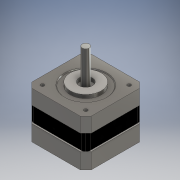
# Autodesk Inventor part: SmallStepper
Saved by Autodesk Inventor 2016 (Build 200138000, 138)
## iProperties
Created: 2016-05-03
Part Number: SmallStepper
Material: Stainless Steel
Document SubType Name: Modeling
Designer: Kurtis
Density: 8 g/cm^3
Appearance: Semi-Polished
Author: Kurtis
Autodesk Inventor part; units mm, degrees
ref_plane "YZ Plane" through (0, 0, 0) normal (1, 0, 0) x (0, 1, 0)
ref_plane "XZ Plane" through (0, 0, 0) normal (0, 1, 0) x (-1, 0, 0)
sketch "Sketch1" plane through (0, 0, 0) normal (0, 0, 1) x (1, 0, 0)
  line L0 (-17.1838, -21) -> (17.1838, -21)
  line L1 (21, -17.1838) -> (21, 17.1838)
  line L2 (17.1838, 21) -> (-17.1838, 21)
  line L3 (-21, 17.1838) -> (-21, -17.1838)
  line L4 (-21, -21) -> (21, 21) construction
  line L5 (21, -21) -> (-21, 21) construction
  line L6 (0, 0) -> (19.0919, -19.0919) construction
  line L7 (0, 0) -> (-19.0919, -19.0919) construction
  line L8 (0, 0) -> (-19.0919, 19.0919) construction
  line L9 (0, 0) -> (19.0919, 19.0919) construction
  line L10 (19.0919, -19.0919) -> (17.1838, -21)
  line L11 (19.0919, -19.0919) -> (21, -17.1838)
  line L12 (-19.0919, -19.0919) -> (-21, -17.1838)
  line L13 (-19.0919, -19.0919) -> (-17.1838, -21)
  line L14 (-19.0919, 19.0919) -> (-21, 17.1838)
  line L15 (-19.0919, 19.0919) -> (-17.1838, 21)
  line L16 (19.0919, 19.0919) -> (21, 17.1838)
  line L17 (19.0919, 19.0919) -> (17.1838, 21)
  line L18 (-15.375, 15.375) -> (15.375, 15.375) construction
  line L19 (15.375, 15.375) -> (15.375, -15.375) construction
  line L20 (15.375, -15.375) -> (-15.375, -15.375) construction
  line L21 (-15.375, -15.375) -> (-15.375, 15.375) construction
  line L22 (-15.375, 15.375) -> (15.375, -15.375) construction
  line L23 (15.375, 15.375) -> (-15.375, -15.375) construction
  circle A0 centre (15.375, 15.375) radius 1.25
  circle A1 centre (-15.375, 15.375) radius 1.25
  circle A2 centre (-15.375, -15.375) radius 1.25
  circle A3 centre (15.375, -15.375) radius 1.25
  dimension "d0" = 42
  dimension "d1" = 42
  dimension "d2" = 27
  dimension "d3" = 27
  dimension "d4" = 27
  dimension "d5" = 27
  dimension "d18" = 34.3675
  dimension "d19" = 30.75
  dimension "d20" = 30.75
  dimension "d21" = 2.5
  dimension "d22" = 2.5
  dimension "d23" = 2.5
  dimension "d24" = 2.5
  constraints: 48 end point, 8 point on line, 6 parallel, 5 perpendicular, 4 centre point, 4 coincident, 4 collinear, 4 midpoint, 2 horizontal
  measures "d0" distance of L5.end L4.end
  measures "d1" distance of L4.end L5.start
  measures "d2" distance of L6.start L6.end
  measures "d3" distance of L6.start L7.end
  measures "d4" distance of L6.start L8.end
  measures "d5" distance of L6.start L9.end
  measures "d18" distance of L2.start L2.end
  measures "d19" distance of L19.end L20.end
  measures "d20" distance of L18.end L19.end
  measures "d21" diameter of A0
  measures "d22" diameter of A1
  measures "d23" diameter of A2
  measures "d24" diameter of A3
extrude "Body" add sketch "Sketch1" along normal blind 33
sketch "Sketch2" plane through (0, 0, 33) normal (0, 0, 1) x (1, 0, 0)
  circle A0 centre (0, 0) radius 11
  dimension "d27" = 22
  constraints: 1 centre point, 1 coincident
  measures "d27" diameter of A0
extrude "Raised" add sketch "Sketch2" along normal blind 2
sketch "Sketch3" plane through (0, 0, 35) normal (0, 0, 1) x (1, 0, 0)
  circle A0 centre (0, 0) radius 2.5
  dimension "d30" = 5
  constraints: 1 centre point, 1 coincident
  measures "d30" diameter of A0
extrude "Axle" add sketch "Sketch3" along normal blind 22
sketch "Sketch4" plane through (0, 0, 35) normal (0, 0, 1) x (1, 0, 0)
  circle A0 centre (0, 0) radius 2.5
  circle A1 centre (0, 0) radius 4.75
  circle A2 centre (0, 0) radius 11
  circle A3 centre (0, 0) radius 15
  dimension "d33" = 9.5
  dimension "d34" = 30
  constraints: 4 centre point, 4 coincident
  measures "d33" diameter of A1
  measures "d34" diameter of A3
extrude "Face Indent" cut sketch "Sketch4" against normal blind 2.5
chamfer "Indent Chamf" distance 0.5 angle 45 1 edges at (-15, 0, 32.5)
sketch "Sketch5" plane through (-17.1838, 21, 0) normal (0, 1, 0) x (1, 0, 0)
  line L0 (17.1838, 0) -> (25.1838, 0)
  line L1 (34.3675, 0) -> (0, 0) projected
  line L2 (25.1838, 0) -> (25.1838, -11.25)
  line L3 (25.1838, -11.25) -> (9.1838, -11.25)
  line L4 (9.1838, -11.25) -> (9.1838, 0)
  line L5 (17.1838, 0) -> (9.1838, 0)
  dimension "d40" = 8
  dimension "d41" = 11.25
  dimension "d42" = 16
  constraints: 10 end point, 3 perpendicular, 2 point on line, 1 collinear
  measures "d40" distance of L0.start L0.end
  measures "d41" distance of L0.end L2.end
  measures "d42" distance of L2.end L3.end
extrude "Power Base" add sketch "Sketch5" along normal blind 3.75
sketch "Sketch6" plane through (-17.1838, 24.75, 0) normal (0, 1, 0) x (1, 0, 0)
  line L0 (25.1838, -11.25) -> (9.1838, -11.25) projected
  line L1 (25.1838, -11.25) -> (25.1838, -4.85)
  line L2 (25.1838, 0) -> (25.1838, -11.25) projected
  line L3 (25.1838, -4.85) -> (9.1838, -4.85)
  line L4 (9.1838, -11.25) -> (9.1838, 0) projected
  line L5 (9.1838, -4.85) -> (9.1838, -11.25)
  line L6 (9.1838, -11.25) -> (25.1838, -11.25)
  line L7 (25.1838, -8.05) -> (24.1838, -8.05) construction
  line L8 (17.1838, -4.85) -> (17.1838, -5.85) construction
  line L9 (9.1838, 0) -> (9.1838, -11.25) construction
  line L10 (9.1838, -8.05) -> (10.1838, -8.05) construction
  line L11 (17.1838, -11.25) -> (17.1838, -10.75) construction
  line L12 (17.1838, -10.75) -> (21.1838, -10.75) construction
  line L13 (17.1838, -10.75) -> (13.1838, -10.75) construction
  line L14 (24.1838, -5.85) -> (10.1838, -5.85)
  line L15 (10.1838, -5.85) -> (10.1838, -10.75)
  line L16 (10.1838, -10.75) -> (13.1838, -10.75)
  line L17 (24.1838, -5.85) -> (24.1838, -10.75)
  line L18 (21.1838, -10.75) -> (24.1838, -10.75)
  line L19 (10.1838, -8.3) -> (24.1838, -8.3) construction
  line L20 (24.1838, -8.3) -> (22.6123, -8.3) construction
  line L21 (22.6123, -8.3) -> (22.1123, -8.3)
  line L22 (22.1123, -8.3) -> (20.5409, -8.3) construction
  line L23 (20.5409, -8.3) -> (20.0409, -8.3)
  line L24 (20.0409, -8.3) -> (18.4695, -8.3) construction
  line L25 (18.4695, -8.3) -> (17.9695, -8.3)
  line L26 (17.9695, -8.3) -> (16.3981, -8.3) construction
  line L27 (16.3981, -8.3) -> (15.8981, -8.3)
  line L28 (15.8981, -8.3) -> (14.3266, -8.3) construction
  line L29 (14.3266, -8.3) -> (13.8266, -8.3)
  line L30 (13.8266, -8.3) -> (12.2552, -8.3) construction
  line L31 (12.2552, -8.3) -> (11.7552, -8.3)
  line L32 (11.7552, -8.3) -> (10.1838, -8.3) construction
  line L33 (22.6123, -8.05) -> (22.1123, -8.05)
  line L34 (22.1123, -8.05) -> (22.1123, -8.55)
  line L35 (22.1123, -8.55) -> (22.6123, -8.55)
  line L36 (22.6123, -8.55) -> (22.6123, -8.05)
  line L37 (22.6123, -8.05) -> (22.1123, -8.55) construction
  line L38 (22.1123, -8.05) -> (22.6123, -8.55) construction
  line L39 (20.5409, -8.05) -> (20.0409, -8.05)
  line L40 (20.0409, -8.05) -> (20.0409, -8.55)
  line L41 (20.0409, -8.55) -> (20.5409, -8.55)
  line L42 (20.5409, -8.55) -> (20.5409, -8.05)
  line L43 (20.5409, -8.05) -> (20.0409, -8.55) construction
  line L44 (20.0409, -8.05) -> (20.5409, -8.55) construction
  line L45 (18.4695, -8.05) -> (17.9695, -8.05)
  line L46 (17.9695, -8.05) -> (17.9695, -8.55)
  line L47 (17.9695, -8.55) -> (18.4695, -8.55)
  line L48 (18.4695, -8.55) -> (18.4695, -8.05)
  line L49 (18.4695, -8.05) -> (17.9695, -8.55) construction
  line L50 (17.9695, -8.05) -> (18.4695, -8.55) construction
  line L51 (16.3981, -8.05) -> (15.8981, -8.05)
  line L52 (15.8981, -8.05) -> (15.8981, -8.55)
  line L53 (15.8981, -8.55) -> (16.3981, -8.55)
  line L54 (16.3981, -8.55) -> (16.3981, -8.05)
  line L55 (16.3981, -8.05) -> (15.8981, -8.55) construction
  line L56 (15.8981, -8.05) -> (16.3981, -8.55) construction
  line L57 (14.3266, -8.05) -> (13.8266, -8.05)
  line L58 (13.8266, -8.05) -> (13.8266, -8.55)
  line L59 (13.8266, -8.55) -> (14.3266, -8.55)
  line L60 (14.3266, -8.55) -> (14.3266, -8.05)
  line L61 (14.3266, -8.05) -> (13.8266, -8.55) construction
  line L62 (13.8266, -8.05) -> (14.3266, -8.55) construction
  line L63 (12.2552, -8.05) -> (11.7552, -8.05)
  line L64 (11.7552, -8.05) -> (11.7552, -8.55)
  line L65 (11.7552, -8.55) -> (12.2552, -8.55)
  line L66 (12.2552, -8.55) -> (12.2552, -8.05)
  line L67 (12.2552, -8.05) -> (11.7552, -8.55) construction
  line L68 (11.7552, -8.05) -> (12.2552, -8.55) construction
  line L69 (13.1838, -10.75) -> (13.1838, -11.25)
  line L70 (21.1838, -10.75) -> (21.1838, -11.25)
  line L71 (9.1838, -11.25) -> (25.1838, -11.25) projected
  point P0 (17.1838, 0)
  point P1 (22.3623, -8.3)
  point P2 (20.2909, -8.3)
  point P3 (18.2195, -8.3)
  point P4 (16.1481, -8.3)
  point P5 (14.0766, -8.3)
  point P6 (12.0052, -8.3)
  dimension "d45" = 6.4
  dimension "d48" = 1
  dimension "d49" = 1
  dimension "d50" = 1
  dimension "d51" = 0.5
  dimension "d52" = 4
  dimension "d53" = 4
  dimension "d59" = 1.5714
  dimension "d60" = 0.5
  dimension "d61" = 1.5714
  dimension "d62" = 0.5
  dimension "d63" = 1.5714
  dimension "d64" = 0.5
  dimension "d65" = 1.5714
  dimension "d66" = 0.5
  dimension "d67" = 1.5714
  dimension "d68" = 0.5
  dimension "d69" = 1.5714
  dimension "d70" = 0.5
  dimension "d71" = 0.5
  dimension "d72" = 0.5
  dimension "d73" = 0.5
  dimension "d74" = 0.5
  dimension "d75" = 0.5
  dimension "d76" = 0.5
  dimension "d77" = 0.5
  dimension "d78" = 0.5
  dimension "d79" = 0.5
  dimension "d80" = 0.5
  dimension "d81" = 2.5714
  dimension "d82" = 3.2
  dimension "d83" = 1
  dimension "d84" = 3.2
  dimension "d85" = 3.2
  constraints: 132 end point, 22 midpoint, 18 parallel, 11 perpendicular, 7 horizontal, 6 point on line, 3 collinear, 3 vertical, 15 other
  measures "d45" distance of L0.start L1.end
  measures "d48" distance of L7.start L7.end
  measures "d49" distance of L8.start L8.end
  measures "d50" distance of L10.start L10.end
  measures "d51" distance of L11.start L11.end
  measures "d52" distance of L11.end L12.end
  measures "d53" distance of L11.end L13.end
  measures "d59" distance of L20.start L20.end
  measures "d60" distance of L20.end L21.end
  measures "d61" distance of L21.end L22.end
  measures "d62" distance of L22.end L23.end
  measures "d63" distance of L23.end L24.end
  measures "d64" distance of L24.end L25.end
  measures "d65" distance of L25.end L26.end
  measures "d66" distance of L26.end L27.end
  measures "d67" distance of L27.end L28.end
  measures "d68" distance of L28.end L29.end
  measures "d69" distance of L29.end L30.end
  measures "d70" distance of L30.end L31.end
  measures "d71" distance of L35.end L34.end
  measures "d72" distance of L34.end L33.end
  measures "d73" distance of L41.end L40.end
  measures "d74" distance of L40.end L39.end
  measures "d75" distance of L47.end L46.end
  measures "d76" distance of L46.end L45.end
  measures "d77" distance of L53.end L52.end
  measures "d78" distance of L52.end L51.end
  measures "d79" distance of L59.end L58.end
  measures "d80" distance of L58.end L57.end
  measures "d81" distance between parallel lines of L2 L36
  measures "d82" distance between parallel lines of L0 L33
  measures "d83" distance between parallel lines of L9 L15
  measures "d84" distance between parallel lines of L7 L0
  measures "d85" distance between parallel lines of L10 L0
extrude "Power Adapter" add sketch "Sketch6" along normal blind 2.25 contours L0 L70 L18 L17 L14 L15 L16 L69 L4 L3 L1 | L36 L35 L34 L21 | L21 L34 L33 L36 | L42 L41 L40 L23 | L23 L40 L39 L42 | L48 L47 L46 L25 | L25 L46 L45 L48 | L54 L53 L52 L27 | L27 L52 L51 L54 | L60 L59 L58 L29 | L29 L58 L57 L60 | L66 L65 L64 L31 | L31 L64 L63 L66
ref_plane "Motor Center" through (0, 0, 16.5) normal (0, 0, 1) x (1, 0, 0)
sketch "Sketch7" plane through (0, 0, 16.5) normal (0, 0, 1) x (1, 0, 0)
  line L0 (-20, 20) -> (20, 20)
  line L1 (20, 20) -> (20, -20)
  line L2 (20, -20) -> (-20, -20)
  line L3 (-20, -20) -> (-20, 20)
  line L4 (-20, 20) -> (20, -20) construction
  line L5 (20, 20) -> (-20, -20) construction
  line L6 (-21, 21) -> (21, 21)
  line L7 (21, 21) -> (21, -21)
  line L8 (21, -21) -> (-21, -21)
  line L9 (-21, -21) -> (-21, 21)
  circle A0 centre (0, 0) radius 4.75 projected
  line L10 (-21, 21) -> (21, -21) construction
  line L11 (21, 21) -> (-21, -21) construction
  dimension "d88" = 40
  dimension "d89" = 40
  dimension "d90" = 42
  dimension "d91" = 42
  constraints: 24 end point, 4 midpoint, 4 parallel, 2 horizontal, 2 perpendicular
  measures "d88" distance of L1.end L2.end
  measures "d89" distance of L0.end L1.end
  measures "d90" distance of L7.end L8.end
  measures "d91" distance of L6.end L7.end
extrude "Coil/Winding" cut sketch "Sketch7" along normal blind 6 and the other way blind 5.25 contours L6 L7 L8 L9
fillet "Cleaner Edges" radius 3 8 edges at (-20, 18.1838, 16.875) (-18.1838, 20, 16.875) (18.1838, 20, 16.875) (20, 18.1838, 16.875) (20, -18.1838, 16.875) (18.1838, -20, 16.875) (-20, -18.1838, 16.875) (-18.1838, -20, 16.875)
sketch "Sketch8" plane through (0, 0, 0) normal (0, 0, -1) x (-1, 0, 0)
  circle A0 centre (0, 0) radius 2.5 projected
  circle A1 centre (0, 0) radius 4.75
  dimension "d97" = 9.5
  constraints: 1 centre point, 1 coincident
  measures "d97" diameter of A1
extrude "Axle Cap" cut sketch "Sketch8" against normal blind 3 contours A0 | A1
chamfer "Cleaner Back Axle" distance 0.5 angle 45 1 edges at (4.75, 0, 3)
body "Solid1"
